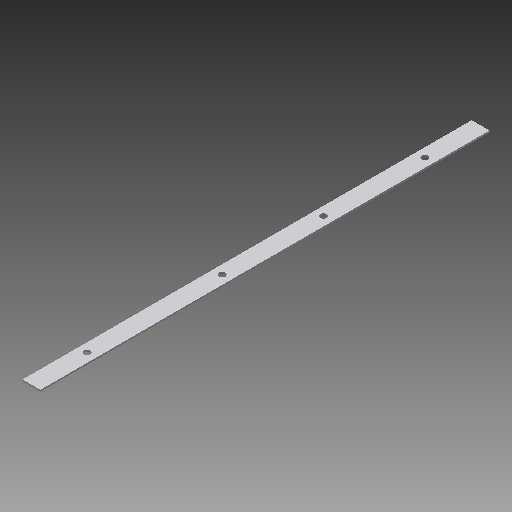
# Autodesk Inventor part: Listwa_oparcia
Saved by Autodesk Inventor 2017 (Build 210142000, 142)
## iProperties
Created: 2015-12-07
Part Number: Listwa_oparcia
Material: Polistyren
Document SubType Name: Modeling
Designer: graaapsik
Density: 1.021 g/cm^3
Appearance: Gładkie - białe
Mass: 9.54278 g
Surface Area: 138.198 cm^2
Volume: 9.3465 cm^3
Author: graaapsik
Autodesk Inventor part; units mm, degrees
ref_plane "YZ Plane" through (0, 0, 0) normal (1, 0, 0) x (0, 1, 0)
ref_plane "XZ Plane" through (0, 0, 0) normal (0, 1, 0) x (-1, 0, 0)
ref_plane "XY Plane" through (0, 0, 0) normal (0, 0, 1) x (1, 0, 0)
sketch "Szkic1" plane through (0, 0, 0) normal (0, 0, 1) x (1, 0, 0)
  line L0 (0, 0) -> (15.9, 0)
  line L1 (15.9, 0) -> (15.9, 1.5)
  line L2 (15.9, 1.5) -> (0, 1.5)
  line L3 (0, 1.5) -> (0, 0)
  dimension "d0" = 15.9
  dimension "d1" = 1.5
  constraints: 8 end point, 2 parallel, 1 horizontal, 1 perpendicular
  measures "d0" distance of L0.start L0.end
  measures "d1" distance of L0.end L1.end
extrude "Wyciągnięcie proste1" add sketch "Szkic1" along normal mid plane 399
sketch "Szkic2" plane through (0, 0, 0) normal (0, 1, 0) x (-1, 0, 0)
  line L0 (0, -199.5) -> (-15.9, -199.5) construction
  line L1 (-7.95, -199.5) -> (-7.95, -178.6885) construction
  line L2 (-15.9, 199.5) -> (0, 199.5) projected
  point P0 (0, 0)
  point P1 (-7.95, -150)
  point P2 (-7.95, -60)
  point P3 (-7.95, 30)
  point P4 (-7.95, 150)
  dimension "d4" = 49.5
  dimension "d5" = 90
  dimension "d6" = 49.5
  dimension "d7" = 90
  constraints: 3 vertical alignment, 2 end point, 1 midpoint, 1 perpendicular, 1 point on line
  measures "d4" distance from line of point (-7.95, -150) L0
  measures "d5" distance of point (-7.95, -60) point (-7.95, -150)
  measures "d6" distance from line of point (-7.95, 150) L2
  measures "d7" distance of point (-7.95, 30) point (-7.95, -60)
hole "Otwór1" at (7.95, 0, -150) at (7.95, 0, -60) at (7.95, 0, 30) at (7.95, 0, 150) direction (0, 1, 0) diameter 6 end through all
